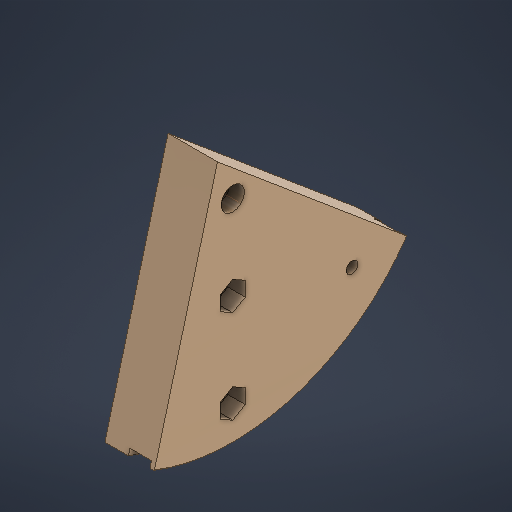
# Autodesk Inventor part: testGT2Pulley_z220
Saved by Autodesk Inventor 2025.2 (Build 292293000, 293)
## iProperties
Created: 2025-05-15
Part Number: testGT2Pulley_z220
Material: Generic
Document SubType Name: Modeling
Designer: Tiago
Density: 1 g/cm^3
Appearance: Brindle
Author: Tiago
Autodesk Inventor part; units mm, degrees
ref_plane "YZ Plane" through (0, 0, 0) normal (1, 0, 0) x (0, 1, 0)
ref_plane "XZ Plane" through (0, 0, 0) normal (0, 1, 0) x (-1, 0, 0)
ref_plane "XY Plane" through (0, 0, 0) normal (0, 0, 1) x (1, 0, 0)
sketch "Sketch1" plane through (0, 0, 0) normal (0, 0, 1) x (1, 0, 0)
  line L0 (0, 4) -> (0, 72.7297)
  line L1 (0, 72.7297) -> (7.1, 72.7297)
  line L2 (7.1, 72.7297) -> (7.1, 69.7722)
  line L3 (7.1, 69.7722) -> (14.5, 69.7722)
  line L4 (14.5, 69.7722) -> (14.5, 72.7297)
  line L5 (14.5, 72.7297) -> (16, 72.7297)
  line L6 (16, 72.7297) -> (16, 4)
  line L7 (16, 0) -> (0, 0)
  line L8 (0, 4) -> (16, 4)
  line L9 (0, 12.5) -> (6, 12.5)
  line L10 (6, 12.5) -> (6, 72.7297)
  line L11 (6, 12.5) -> (6, 4)
  line L12 (14.5, 72.7297) -> (14.5, 4)
  dimension "L" = 16
  dimension "d1" = 7.1
  dimension "DE" = 145.4594
  dimension "d3" = 139.5444
  dimension "d4" = 7.4
  dimension "d5" = 145.4594
  dimension "Bore" = 8
  dimension "d33" = 25
  dimension "d34" = 6
  constraints: 26 end point, 10 perpendicular, 4 point on line, 2 horizontal, 2 vertical alignment, 1 vertical
  measures "L" distance of L7.start L7.end
  measures "d1" distance between parallel lines of L0 L2
  measures "DE" diameter of L1 L7
  measures "d3" diameter of L3 L7
  measures "d4" distance between parallel lines of L4 L2
  measures "d5" diameter of L5 L7
  measures "Bore" diameter of L8 L7
  measures "d33" diameter of L9 L7
  measures "d34" distance of L9.start L9.end
revolve "Revolution1" add sketch "Sketch1" angle 360 about axis through (16, 0, 0) along (-1, 0, 0) contours L11 L10 L1 L2 L3 L12 L8 | L12 L4 L5 L6 L8
sketch "Sketch3" plane through (7.1, 0, 0) normal (1, 0, 0) x (0, 0, -1)
  line L0 (0, 0) -> (0, 8.9731) construction
  line L1 (0, 0) -> (0.1349, 9.4467) construction
  line L2 (0, 0) -> (0.1914, 9.5743) construction
  line L3 (0, 0) -> (0.266, 9.3119) construction
  circle A0 centre (0, 0) radius 69.7722
  circle A1 centre (0, 0) radius 70.3272 construction
  arc A2 (1.4824, 70.4759) -> (1.3431, 70.6738) centre (1.3402, 70.5238) ccw
  arc A3 (1.4824, 70.4759) -> (1.9924, 69.7437) centre (2.0083, 70.2985) ccw
  arc A4 (0.6756, 70.6833) -> (0.5307, 70.4895) centre (0.6742, 70.5333) ccw
  arc A5 (0, 69.7722) -> (0.5307, 70.4895) centre (0, 70.3272) ccw
  circle A6 centre (0, 0.0002) radius 70.0282 construction
  arc A7 (1.3431, 70.6738) -> (0.6756, 70.6833) centre (0, 0) ccw
  point P0 (0, 69.7722)
  dimension "di" = 139.5444
  dimension "d12" = 0.555
  dimension "d8" = 0.818
  dimension "ANGLEP" = 1.636
  dimension "d10" = 0.327
  dimension "d16" = 0.3
  dimension "d17" = 0.555
  dimension "d18" = 0.15
  dimension "PD" = 140.0564
  constraints: 10 point on circle, 8 end point, 6 centre point, 5 symmetric about line, 2 tangent, 1 coincident, 1 point on line, 1 vertical, 8 other
  measures "d8" angle of L0 L1
  measures "ANGLEP" angle of L0 L3
  measures "d10" angle of L1 L2
  measures "d16" diameter of A2
  measures "d17" radius of A3
  measures "d18" radius of A2
  measures "PD" diameter of A6
extrude "Extrusion2" add sketch "Sketch3" along normal up to surface (7.4 mm away) contours A0 A5 A4 A7 A2 A3
pattern_circular "Circular Pattern2" count 220 over 360 about axis through (-10, 0, 0) along (1, 0, 0) of "Extrusion2"
sketch "Sketch6" plane through (6, 0, 0) normal (-1, 0, 0) x (0, 0, 1)
  circle A0 centre (0, 0) radius 4.5
  line L0 (0, -41) -> (0, 41) construction
  line L1 (-41, 0) -> (41, 0) construction
  circle A1 centre (41, -41) radius 2
  line L2 (0, 0) -> (0, -45) construction
  circle A2 centre (0, 0) radius 65 construction
  line L3 (46, -41) -> (36, -41) construction
  line L4 (41, -36) -> (41, -46) construction
  line L5 (46, -41) -> (46, -45.9239) construction
  line L6 (45.9239, -46) -> (41, -46) construction
  line L7 (36, -41) -> (36, -46) construction
  line L8 (36, -46) -> (41, -46) construction
  line L9 (46, -41) -> (46, -36) construction
  line L10 (46, -36) -> (41, -36) construction
  line L11 (39, -36) -> (41, -36) construction
  line L12 (36, -41) -> (36, -39) construction
  line L13 (46, -36) -> (51.1878, -40.06) construction
  arc A3 (39, -36) -> (36, -39) centre (39, -39) ccw construction
  line L14 (46, -46) -> (36, -36) construction
  line L15 (36, -46) -> (40.06, -51.1878) construction
  circle A4 centre (0, -45) radius 5.75
  line L16 (0, -61) -> (0, -29) construction
  circle A5 centre (0, -29) radius 2.25
  circle A6 centre (0, -61) radius 2.25
  circle A7 centre (52.8275, 30.5) radius 2.25
  circle A8 centre (38.9711, 22.5) radius 5.75
  circle A9 centre (25.1147, 14.5) radius 2.25
  circle A10 centre (-52.8275, 30.5) radius 2.25
  circle A11 centre (-38.9711, 22.5) radius 5.75
  circle A12 centre (-25.1147, 14.5) radius 2.25
  circle A13 centre (41, 41) radius 2
  line L17 (46, 41) -> (36, 41) construction
  line L18 (41, 36) -> (41, 46) construction
  line L19 (46, 41) -> (46, 45.9239) construction
  line L20 (45.9239, 46) -> (41, 46) construction
  line L21 (36, 46) -> (41, 46) construction
  line L22 (36, 41) -> (36, 46) construction
  line L23 (39, 36) -> (41, 36) construction
  line L24 (36, 41) -> (36, 39) construction
  line L25 (46, 36) -> (41, 36) construction
  line L26 (46, 41) -> (46, 36) construction
  line L27 (46, 36) -> (51.1878, 40.06) construction
  arc A14 (36, 39) -> (39, 36) centre (39, 39) ccw construction
  line L28 (46, 46) -> (36, 36) construction
  line L29 (36, 46) -> (40.06, 51.1878) construction
  circle A15 centre (-41, -41) radius 2
  line L30 (-46, -41) -> (-36, -41) construction
  line L31 (-41, -36) -> (-41, -46) construction
  line L32 (-46, -41) -> (-46, -45.9239) construction
  line L33 (-45.9239, -46) -> (-41, -46) construction
  line L34 (-36, -46) -> (-41, -46) construction
  line L35 (-36, -41) -> (-36, -46) construction
  line L36 (-39, -36) -> (-41, -36) construction
  line L37 (-36, -41) -> (-36, -39) construction
  line L38 (-46, -36) -> (-41, -36) construction
  line L39 (-46, -41) -> (-46, -36) construction
  line L40 (-46, -36) -> (-51.1878, -40.06) construction
  arc A16 (-36, -39) -> (-39, -36) centre (-39, -39) ccw construction
  line L41 (-46, -46) -> (-36, -36) construction
  line L42 (-36, -46) -> (-40.06, -51.1878) construction
  line L43 (-36, 46) -> (-40.06, 51.1878) construction
  line L44 (-36, 46) -> (-41, 46) construction
  line L45 (-36, 41) -> (-36, 46) construction
  line L46 (-45.9239, 46) -> (-41, 46) construction
  line L47 (-36, 41) -> (-36, 39) construction
  line L48 (-46, 41) -> (-46, 45.9239) construction
  line L49 (-46, 41) -> (-36, 41) construction
  arc A17 (-39, 36) -> (-36, 39) centre (-39, 39) ccw construction
  line L50 (-46, 46) -> (-36, 36) construction
  line L51 (-41, 36) -> (-41, 46) construction
  line L52 (-39, 36) -> (-41, 36) construction
  line L53 (-46, 36) -> (-41, 36) construction
  line L54 (-46, 41) -> (-46, 36) construction
  line L55 (-46, 36) -> (-51.1878, 40.06) construction
  circle A18 centre (-41, 41) radius 2
  line L56 (0, 65) -> (0, 53) construction
  arc A19 (-11.9488, 63.8923) -> (11.9488, 63.8923) centre (0, 65) ccw
  circle A20 centre (-18.25, 0) radius 2.25
  circle A21 centre (18.25, 0) radius 2.25
  circle A22 centre (0, 0) radius 72.7297
  point P0 (43.5, -36)
  point P1 (36.8787, -36.8787)
  point P2 (43.5, 36)
  point P3 (36.8787, 36.8787)
  point P4 (-43.5, -36)
  point P5 (-36.8787, -36.8787)
  point P6 (-36.8787, 36.8787)
  point P7 (-43.5, 36)
  point P8 (0, 53)
  dimension "d43" = 9
  dimension "d45" = 82
  dimension "d46" = 82
  dimension "d48" = 45
  dimension "d60" = 130
  dimension "d71" = 10
  dimension "d72" = 10
  dimension "d73" = 5
  dimension "d74" = 3
  dimension "d125" = 4.9238
  dimension "d126" = 41
  dimension "d127" = 41
  dimension "d128" = 5
  dimension "d129" = 5
  dimension "d131" = 4
  dimension "d132" = 11.5
  dimension "d134" = 32
  dimension "d135" = 4.5
  dimension "d136" = 4.5
  dimension "d139" = 360
  dimension "d145" = 13.906
  dimension "d146" = 90
  dimension "d147" = 90
  dimension "d157" = 12
  dimension "d158" = 12
  dimension "d159" = 12
  dimension "d160" = 53
  dimension "d184" = 4.5
  dimension "d185" = 4.5
  dimension "d186" = 18.25
  dimension "d187" = 18.25
  dimension "d193" = 145.4594
  constraints: 114 end point, 61 symmetric about line, 23 centre point, 19 point on circle, 14 coincident, 12 point on line, 8 midpoint, 3 horizontal alignment, 3 vertical, 2 line through centre, 2 perpendicular, 2 tangent, 1 horizontal, 26 other
  measures "d43" diameter of A0
  measures "d45" distance of L0.start L0.end
  measures "d46" distance of L1.start L1.end
  measures "d48" distance of L2.start L2.end
  measures "d60" diameter of A2
  measures "d71" distance of L3.start L3.end
  measures "d72" distance of L4.start L4.end
  measures "d73" distance of L3.start L14.start
  measures "d74" radius of A3
  measures "d125" distance of L6.start L4.end
  measures "d126" distance from line of L1 A1.centre
  measures "d127" distance from line of L0 point (41, -41)
  measures "d128" horizontal distance of L14.start A1.centre
  measures "d129" horizontal distance of L14.start A1.centre
  measures "d131" diameter of A1
  measures "d132" diameter of A4
  measures "d134" distance of L16.start L16.end
  measures "d135" diameter of A5
  measures "d136" diameter of A6
  measures "d145" angle of L13 L15
  measures "d146" angle of L3 L12
  measures "d147" angle of L3 L7
  measures "d157" distance of L56.start L56.end
  measures "d158" radius of A19
  measures "d159" distance of point (0, 53) L56.start
  measures "d160" distance of point (0, 0) point (0, 53)
  measures "d184" diameter of A21
  measures "d185" diameter of A20
  measures "d186" distance of point (0, 0) A21.centre
  measures "d187" distance of point (0, 0) A20.centre
  measures "d193" diameter of A22
sketch "Sketch8" plane through (16, 0, 0) normal (1, 0, 0) x (0, 0, -1)
  line L0 (0, 0) -> (0, -69)
  line L1 (-1.25, -71.25) -> (1.25, -71.25)
  line L2 (1.25, -71.25) -> (1.25, -66.75)
  line L3 (1.25, -66.75) -> (-1.25, -66.75)
  line L4 (-1.25, -66.75) -> (-1.25, -71.25)
  line L5 (-1.25, -71.25) -> (1.25, -66.75) construction
  line L6 (1.25, -71.25) -> (-1.25, -66.75) construction
  dimension "d107" = 69
  dimension "d108" = 4.5
  dimension "d109" = 2.5
  constraints: 14 end point, 2 midpoint, 2 parallel, 1 horizontal, 1 perpendicular, 1 vertical
  measures "d107" distance of L0.start L0.end
  measures "d108" distance of L1.end L2.end
  measures "d109" distance of L1.start L1.end
extrude "Extrusion16" cut sketch "Sketch6" along normal mid plane 30 contours A1 | A4 | A5 | A6 | A7 | A8 | A9 | A10 | A11 | A12 | A13 | A15 | A18 | A20 | A21
extrude "Extrusion17" add sketch "Sketch8" along normal blind 5
fillet "Fillet9" radius 0.5 2 edges at (21, -71.25, 0) (21, -66.75, 0)
extrude "Extrusion18" add sketch "Sketch6" along normal blind 7
fillet "Fillet10" radius 0.2 2 edges at (16, -72.7297, 0) (-1, 0, -72.7297)
sketch "Sketch14" plane through (16, 0, 0) normal (1, 0, 0) x (0, 0, -1)
  circle A0 centre (-25.1147, 14.5) radius 2.25 projected
  circle A1 centre (-52.8275, 30.5) radius 2.25 projected
  circle A2 centre (25.1147, 14.5) radius 2.25 projected
  circle A3 centre (52.8275, 30.5) radius 2.25 projected
  circle A4 centre (18.25, 0) radius 2.25 projected
  circle A5 centre (-18.25, 0) radius 2.25 projected
  circle A6 centre (0, -29) radius 2.25 projected
  circle A7 centre (0, -61) radius 2.25 projected
  circle A8 centre (-25.1147, 14.5) radius 2.25
  circle A9 centre (-52.8275, 30.5) radius 2.25
  circle A10 centre (25.1147, 14.5) radius 2.25
  circle A11 centre (52.8275, 30.5) radius 2.25
  circle A12 centre (18.25, 0) radius 2.25
  circle A13 centre (-18.25, 0) radius 2.25
  circle A14 centre (0, -29) radius 2.25
  circle A15 centre (0, -61) radius 2.25
  line L0 (0, -24) -> (4.3301, -26.5)
  line L1 (4.3301, -26.5) -> (4.3301, -31.5)
  line L2 (4.3301, -31.5) -> (0, -34)
  line L3 (0, -34) -> (-4.3301, -31.5)
  line L4 (-4.3301, -31.5) -> (-4.3301, -26.5)
  line L5 (-4.3301, -26.5) -> (0, -24)
  line L6 (0, -56) -> (4.3301, -58.5)
  line L7 (4.3301, -58.5) -> (4.3301, -63.5)
  line L8 (4.3301, -63.5) -> (0, -66)
  line L9 (0, -66) -> (-4.3301, -63.5)
  line L10 (-4.3301, -63.5) -> (-4.3301, -58.5)
  line L11 (-4.3301, -58.5) -> (0, -56)
  line L12 (18.25, 5) -> (22.5801, 2.5)
  line L13 (22.5801, 2.5) -> (22.5801, -2.5)
  line L14 (22.5801, -2.5) -> (18.25, -5)
  line L15 (18.25, -5) -> (13.9199, -2.5)
  line L16 (13.9199, -2.5) -> (13.9199, 2.5)
  line L17 (13.9199, 2.5) -> (18.25, 5)
  line L18 (-18.25, 5) -> (-13.9199, 2.5)
  line L19 (-13.9199, 2.5) -> (-13.9199, -2.5)
  line L20 (-13.9199, -2.5) -> (-18.25, -5)
  line L21 (-18.25, -5) -> (-22.5801, -2.5)
  line L22 (-22.5801, -2.5) -> (-22.5801, 2.5)
  line L23 (-22.5801, 2.5) -> (-18.25, 5)
  line L24 (48.4974, 28) -> (48.4974, 33)
  line L25 (57.1577, 28) -> (52.8275, 25.5)
  line L26 (48.4974, 33) -> (52.8275, 35.5)
  line L27 (57.1577, 33) -> (57.1577, 28)
  line L28 (52.8275, 35.5) -> (57.1577, 33)
  line L29 (52.8275, 25.5) -> (48.4974, 28)
  line L30 (20.7846, 12) -> (20.7846, 17)
  line L31 (20.7846, 17) -> (25.1147, 19.5)
  line L32 (25.1147, 9.5) -> (20.7846, 12)
  line L33 (25.1147, 19.5) -> (29.4449, 17)
  line L34 (29.4449, 12) -> (25.1147, 9.5)
  line L35 (29.4449, 17) -> (29.4449, 12)
  line L36 (-48.4974, 28) -> (-52.8275, 25.5)
  line L37 (-52.8275, 35.5) -> (-48.4974, 33)
  line L38 (-52.8275, 25.5) -> (-57.1577, 28)
  line L39 (-57.1577, 33) -> (-52.8275, 35.5)
  line L40 (-57.1577, 28) -> (-57.1577, 33)
  line L41 (-48.4974, 33) -> (-48.4974, 28)
  line L42 (-20.7846, 12) -> (-25.1147, 9.5)
  line L43 (-25.1147, 9.5) -> (-29.4449, 12)
  line L44 (-20.7846, 17) -> (-20.7846, 12)
  line L45 (-29.4449, 12) -> (-29.4449, 17)
  line L46 (-25.1147, 19.5) -> (-20.7846, 17)
  line L47 (-29.4449, 17) -> (-25.1147, 19.5)
  point P0 (0, 0)
  point P1 (52.8275, 30.5)
  point P2 (52.8275, 30.5)
  point P3 (25.1147, 14.5)
  point P4 (25.1147, 14.5)
  point P5 (-52.8275, 30.5)
  point P6 (-52.8275, 30.5)
  point P7 (-25.1147, 14.5)
  point P8 (-25.1147, 14.5)
  dimension "d197" = 10
  dimension "d198" = 10
  dimension "d199" = 10
  dimension "d200" = 10
  dimension "d203" = 360
  constraints: 96 end point, 16 coincident, 8 centre point, 8 concentric, 4 vertical alignment, 137 other
  measures "d197" distance of L0.start L2.end
  measures "d198" distance of L8.end L6.start
  measures "d199" distance of L12.start L14.end
  measures "d200" distance of L18.start L20.end
extrude "Extrusion19" cut sketch "Sketch14" against normal blind 6
extrude "Extrusion20" add sketch "Sketch6" against normal up to surface (10 mm away) contours A4 | A8 | A11
extrude "Extrusion21" cut sketch "Sketch6" against normal blind 5 contours A0 | A4 | A8 | A11
sketch "Sketch15" plane through (16, 0, 0) normal (1, 0, 0) x (0, 0, -1)
  line L0 (-5.2313, 13.5487) -> (-35.1056, -97.9437)
  line L1 (-5.2313, 13.5487) -> (-5.2313, -51.5155) construction
  line L2 (-5.2313, 13.5487) -> (88.3293, -64.958)
  line L3 (88.3293, -64.958) -> (-35.1056, -97.9437)
  point P0 (0, 0)
  dimension "d211" = 15
  dimension "d212" = 65
  dimension "d216" = 100
  dimension "d219" = 13.5487
  dimension "d220" = 5.2313
  dimension "d221" = 127.7664
  constraints: 8 end point, 1 vertical
  measures "d211" angle of L0 L1
  measures "d212" angle of L0 L2
  measures "d216" distance from line of L0.start L3
  measures "d219" vertical distance of L0.start point (0, 0)
  measures "d220" horizontal distance of L0.start point (0, 0)
  measures "d221" distance of L2.end L0.end
extrude "Extrusion22" cut sketch "Sketch15" against normal blind 30 keep common part
equation "\"d3\" = di"
equation "\"d5\" = DE"
equation "\"d8\" = 0.5 * ANGLEP"
equation "\"d10\" = 0.2 * ANGLEP"
equation "\"PD\" = 0.63662 * zz"
equation "\"d46\" = d45"
equation "\"d52\" = 5.5"
equation "\"d59\" = 5.5"
equation "\"zz\" = 220"
body "Solid1"
